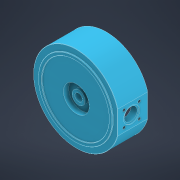
# Autodesk Inventor part: 008
Saved by Autodesk Inventor 2022 (Build 260153000, 153)
## iProperties
Created: 2021-11-17
Part Number: 008
Material: Steel, Carbon
Document SubType Name: Modeling
Designer: vinicius.miguel
Density: 7.85 g/cm^3
Appearance: Turquoise
Mass: 475.252 g
Surface Area: 233.832 cm^2
Volume: 60.5416 cm^3
Author: vinicius.miguel
Autodesk Inventor part; units mm, degrees
ref_plane "XZ Plane" through (0, 0, 0) normal (0, 1, 0) x (-1, 0, 0)
ref_plane "XY Plane" through (0, 0, 0) normal (0, 0, 1) x (1, 0, 0)
sketch "Sketch1" plane through (0, 0, 0) normal (0, 1, 0) x (-1, 0, 0)
  line L0 (0, 0) -> (0, 28)
  line L1 (-3.5, 20) -> (-15, 20)
  line L2 (-15, 20) -> (-15, 25)
  line L3 (-15, 25) -> (-32, 25)
  line L4 (-32, 25) -> (-32, 0)
  line L5 (-32, 0) -> (-40, 0)
  line L6 (-40, 0) -> (-40, 28)
  line L7 (-40, 28) -> (-34.5, 28)
  line L8 (-34.5, 28) -> (-34.5, 29)
  line L9 (-34.5, 29) -> (-31.5, 29)
  line L10 (-31.5, 29) -> (-31.5, 28)
  line L11 (-31.5, 28) -> (-12, 28)
  line L12 (-12, 23) -> (-3.5, 23)
  line L13 (-12, 28) -> (-12, 23)
  line L14 (-3.5, 23) -> (-3.5, 20)
  line L15 (-3.5, 23) -> (-3.5, 26)
  line L16 (-3.5, 26) -> (-6, 26)
  line L17 (-6, 26) -> (-6, 23)
  dimension "d5" = 69
  dimension "d6" = 3
  dimension "d7" = 1
  dimension "d8" = 80
  dimension "d10" = 3
  dimension "d11" = 5
  dimension "d12" = 30
  dimension "d37" = 8
  dimension "d64" = 28
  dimension "d74" = 7
  dimension "d75" = 24
  dimension "d76" = 3
  dimension "d77" = 2.5
  dimension "d78" = 3
  constraints: 36 end point, 16 perpendicular, 4 vertical, 2 horizontal alignment, 2 point on line
  measures "d5" diameter of L8 L0
  measures "d6" distance of L8.end L9.end
  measures "d7" distance of L9.end L10.end
  measures "d8" diameter of L6 L0
  measures "d10" distance between parallel lines of L11 L3
  measures "d11" distance of L1.end L2.end
  measures "d12" diameter of L2 L0
  measures "d37" distance between parallel lines of L6 L4
  measures "d64" distance of L5.end L6.end
  measures "d74" diameter of L14 L0
  measures "d75" diameter of L13 L0
  measures "d76" distance of L12.end L1.start
  measures "d77" distance of L15.end L16.end
  measures "d78" distance of L16.end L17.end
revolve "Revolution1" add sketch "Sketch1" angle 360 about axis through (0, 0, 0) along (0, 0, 1)
ref_plane "Work Plane1" through (40, 0, 14) normal (1, 0, 0) x (0, 1, 0)
sketch "Sketch7" plane through (40, 0, 14) normal (1, 0, 0) x (0, 1, 0)
  line L0 (32, 11) -> (-32, 11) projected
  line L1 (32, -14) -> (-32, -14) projected
  line L2 (32, 11) -> (-32, 11) projected
  line L3 (0, 11) -> (0, -14) construction
  line L4 (21.032, 28.35) -> (-21.032, 28.35)
  line L5 (-21.032, 28.35) -> (-21.032, -31.35)
  line L6 (-21.032, -31.35) -> (21.032, -31.35)
  line L7 (21.032, -31.35) -> (21.032, 28.35)
  line L8 (21.032, 28.35) -> (-21.032, -31.35) construction
  line L9 (-21.032, 28.35) -> (21.032, -31.35) construction
  point P0 (0, -1.5)
  constraints: 14 end point, 4 midpoint, 2 parallel, 2 perpendicular, 1 horizontal
extrude "Extrusion5" cut sketch "Sketch7" against normal blind 1.5
chamfer "Chamfer1" distance 0.25 angle 45 4 edges at (-40, 0, 28) (-34.5, 0, 29) (-31.5, 0, 29) (38.5, 0, 28)
sketch "Sketch8" plane through (38.5, 0, 14) normal (1, 0, 0) x (0, 0, -1)
  circle A0 centre (-1, 0) radius 6
  line L0 (14, 40) -> (14, -40) projected
  line L1 (-14, -39.75) -> (-14, 39.75) projected
  point P0 (14, 0)
  point P1 (14, 10.8513)
  point P2 (14, -10.8513)
  point P3 (-14, -10.8167)
  point P4 (-14, 10.8167)
  point P5 (14, 0)
  dimension "d44" = 12
  dimension "d66" = 13
  constraints: 1 centre point, 1 horizontal alignment, 1 midpoint
  measures "d44" diameter of A0
  measures "d66" distance from line of L1 A0.centre
extrude "Extrusion6" cut sketch "Sketch8" against normal blind 20
sketch "Sketch10" plane through (38.5, 0, 14) normal (1, 0, 0) x (0, 0, -1)
  circle A0 centre (-1, 0) radius 6 projected
  line L0 (-1, 0) -> (14, 0)
  line L1 (14, 10.8513) -> (14, -10.8513) projected
  line L2 (-1, 0) -> (6.0711, 7.0711)
  point P0 (14, 0)
  dimension "d51" = 10
  dimension "d65" = 45
  constraints: 4 end point, 1 horizontal, 1 midpoint
  measures "d51" distance of L2.end L0.start
  measures "d65" angle of L0 L2
hole "Hole2" at (38.5, 7.0711, 7.9289) direction (-1, 0, 0) diameter 2.459 depth 4.5 tip angle 118 thread size "M3x0.5" class "6H" standard "ISO Metric profile"
pattern_circular "Circular Pattern1" count 4 over 360 about axis through (38.5, 0, 15) along (-1, 0, 0) of "Hole2"
sketch "Sketch11" plane through (38.5, 0, 14) normal (1, 0, 0) x (0, 0, -1)
  circle A0 centre (-1, 0) radius 6 projected
  circle A1 centre (-1, 0) radius 7.5
  point P0 (14, 0)
  dimension "d70" = 12
  dimension "d71" = 1.5
  constraints: 1 centre point
  measures "d70" diameter of A0
  measures "d71" radial gap between concentric circles of A0 A1
extrude "Extrusion8" cut sketch "Sketch11" against normal blind 0.75
body "Solid1"
